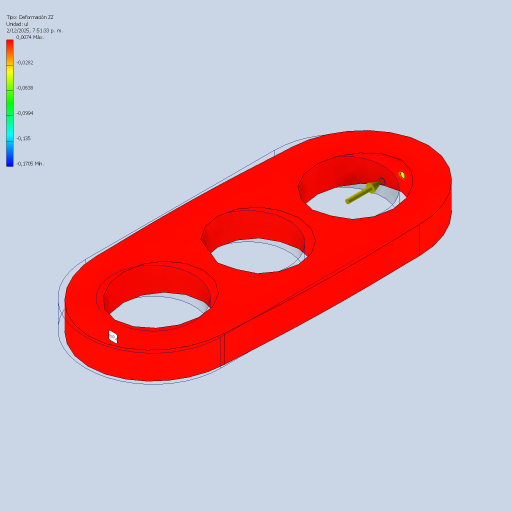
# Autodesk Inventor part: mod3
Saved by Autodesk Inventor 2024 (Build 280153000, 153)
## iProperties
Created: 2025-12-02
Part Number: mod3
Material: Aluminio 6061
Document SubType Name: Modeling
Designer: ANDRES
Density: 2.7 g/cm^3
Appearance: Aluminio - Plano
Author: ANDRES
## iProperties of the stored document mod3_3DPrint.ipt
Created: 2025-12-02
Part Number: mod3_3DPrint
Material: Genérico
Document SubType Name: Modeling
Designer: ANDRES
Density: 1 g/cm^3
Appearance: Valor por defecto
Author: ANDRES
Autodesk Inventor part; units mm, degrees
sketch "Boceto1" plane through (0, 0, 0) normal (0, 1, 0) x (-1, 0, 0)
  line L0 (0, 35) -> (0, -35) construction
  line L1 (25, 35) -> (25, -35)
  line L2 (-25, -35) -> (-25, 35)
  arc A0 (25, 35) -> (-25, 35) centre (0, 35) ccw
  arc A1 (-25, -35) -> (25, -35) centre (0, -35) ccw
  circle A2 centre (0, -35) radius 15
  circle A3 centre (0, 35) radius 15
  line L3 (0, -20) -> (0, -20)
  line L4 (15, -35) -> (-15, -35)
  line L5 (94.5074, 0) -> (-76.0102, 0) construction
  line L6 (15, 35) -> (-15, 35)
  line L7 (15, -35) -> (-15, -35)
  circle A4 centre (0, 0) radius 15
  point P0 (0, 60)
  point P1 (0, -60)
  point P2 (0, -20)
  point P3 (15, 35)
  dimension "largo" = 120
  dimension "ancho" = 50
  dimension "espesor_junta" = 10
  dimension "d3" = 10
  dimension "d6" = 0
  dimension "d12" = 30
  constraints: 18 end point, 10 point on circle, 5 centre point, 4 tangent, 3 horizontal, 3 midpoint, 2 concentric, 2 symmetric about line, 2 vertical, 1 coincident, 1 parallel, 1 vertical alignment
  measures "largo" distance of point (0, 60) point (0, -60)
  measures "ancho" distance between parallel lines of L2 L1
  measures "espesor_junta" radial gap between concentric circles of A1 A2
  measures "d3" radial gap between concentric circles of A0 A3
  measures "d6" distance of L3.start L3.end
  measures "d12" diameter of A4
extrude "Extrusión3" add sketch "Boceto1" along normal blind 10
ref_plane "Plano de trabajo1" through (0, 0, 35) normal (1, 0, 0) x (0, 0, -1)
sketch "Boceto2" plane through (0, 0, 35) normal (1, 0, 0) x (0, 0, -1)
  line L0 (15, 0) -> (15, 10) projected
  line L1 (15, 10) -> (20, 10) projected
  line L2 (20, 10) -> (20, 0) projected
  line L3 (20, 0) -> (15, 0) projected
  line L4 (55, 10) -> (55, 0) projected
  line L5 (55, 0) -> (50, 0) projected
  line L6 (50, 0) -> (50, 10) projected
  line L7 (50, 10) -> (55, 10) projected
  line L8 (95, 10) -> (95, 0) projected
  line L9 (95, 0) -> (85, 0) projected
  line L10 (85, 0) -> (85, 10) projected
  line L11 (85, 10) -> (95, 10) projected
  line L12 (-25, 0) -> (-25, 10) projected
  line L13 (-25, 10) -> (-15, 10) projected
  line L14 (-15, 10) -> (-15, 0) projected
  line L15 (-15, 0) -> (-25, 0) projected
  line L16 (-15, 10) -> (-15, 0) projected
  point P0 (35, 0)
  point P1 (85, 5)
  point P2 (-15, 5)
  constraints: 2 midpoint
ref_plane "Plano de trabajo2" through (0, 5, -50) normal (0, 0, 1) x (1, 0, 0)
ref_plane "Plano de trabajo3" through (0, 10, 50) normal (0, 0, 1) x (1, 0, 0)
sketch "Boceto3" plane through (0, 5, -50) normal (0, 0, 1) x (1, 0, 0)
  circle A0 centre (0, 0) radius 1
  point P0 (0, -5)
  dimension "d16" = 2
  constraints: 1 centre point
  measures "d16" diameter of A0
extrude "Extrusión4" add sketch "Boceto3" along normal blind 0.1
sketch "Boceto4" plane through (0, 10, 50) normal (0, 0, 1) x (1, 0, 0)
  line L0 (-20, -10) -> (-20, 0) projected
  line L1 (-20, 0) -> (0, 0) projected
  line L2 (0, 0) -> (0, -10) projected
  line L3 (20, -10) -> (0, -10) projected
  line L4 (20, 0) -> (20, -10) projected
  line L5 (0, 0) -> (20, 0) projected
  line L6 (0, -10) -> (-20, -10) projected
  circle A0 centre (0, -5) radius 1
  dimension "d19" = 2
  constraints: 1 centre point, 1 midpoint
  measures "d19" diameter of A0
extrude "Extrusión5" add sketch "Boceto4" against normal blind 0.1 contours A0 L2 | L2 A0
equation "\"d3\" = espesor_junta"
equation "\"d15\" = -0.5 * ancho"
